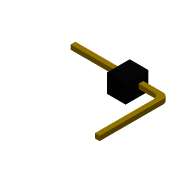
# Autodesk Inventor part: HeaderRight1
Saved by Autodesk Inventor 2015 (Build 190159000, 159)
## iProperties
Created: 2014-08-02
Part Number: HeaderRight1
Material: Generic
Document SubType Name: Modeling
Designer: david
Density: 1 g/cm^3
Appearance: Black
Author: david
Autodesk Inventor part; units mm, degrees
ref_plane "YZ Plane" through (0, 0, 0) normal (1, 0, 0) x (0, 1, 0)
ref_plane "XZ Plane" through (0, 0, 0) normal (0, 1, 0) x (-1, 0, 0)
sketch "Sketch1" plane through (0, 0, 0) normal (0, 1, 0) x (-1, 0, 0)
  line L0 (2.5467, 7.6401) -> (1.9117, 7.6401)
  line L1 (1.9117, 7.6401) -> (1.9117, -1.0276)
  line L2 (2.7055, -1.8214) -> (14.6752, -1.8214)
  line L3 (14.6752, -1.8214) -> (14.6752, -1.1864)
  line L4 (14.6752, -1.1864) -> (3.3405, -1.1864)
  line L5 (2.5467, 7.6401) -> (2.5467, -0.3926)
  line L6 (14.6752, -1.5039) -> (20.4389, -1.5039) construction
  line L7 (2.2292, 7.6401) -> (2.2292, 18.3973) construction
  line L8 (8.8332, 0.2741) -> (6.2932, 0.2741) construction
  line L9 (6.2932, 0.2741) -> (6.2932, -2.8247) construction
  line L10 (8.8332, -2.8247) -> (8.8332, 0.2741) construction
  arc A0 (2.5467, -0.3926) -> (3.3405, -1.1864) centre (3.3405, -0.3926) ccw
  arc A1 (1.9117, -1.0276) -> (2.7055, -1.8214) centre (2.7055, -1.0276) ccw
  line L11 (8.8332, -2.8247) -> (6.2932, -2.8247) construction
  dimension "d2" = 0.635
  dimension "d7" = 3.0988
  dimension "d9" = 1.778
  dimension "d10" = 7.366
  dimension "d11" = 4.064
  dimension "d12" = 5.842
  dimension "d13" = 0.7937
  constraints: 24 end point, 6 perpendicular, 4 horizontal, 4 point on circle, 4 tangent, 2 centre point, 2 midpoint, 2 vertical, 1 equal radius, 1 parallel
  measures "d2" distance of L0.start L0.end
  measures "d7" distance of L10.start L8.start
  measures "d9" distance between parallel lines of L8 L6
  measures "d10" distance between parallel lines of L8 L0
  measures "d11" distance between parallel lines of L9 L7
  measures "d12" distance between parallel lines of L10 L3
  measures "d13" radius of A0
extrude "Extrusion1" add sketch "Sketch1" along normal mid plane 0.635
ref_plane "Work Plane1" through (-5.4042, -0.3175, 7.6401) normal (-1, 0, 0) x (0, 0, 1)
sketch "Sketch2" plane through (-5.4042, -0.3175, 7.6401) normal (-1, 0, 0) x (0, 0, 1)
  line L0 (-8.8265, 0) -> (-8.8265, 0.635) projected
  line L1 (-9.4615, 0.635) -> (-8.8265, 0.635) projected
  line L2 (-9.4615, 0) -> (-9.4615, 0.635) projected
  line L3 (-8.8265, 0) -> (-9.4615, 0) projected
  line L4 (-7.0485, -0.9525) -> (-10.1473, -0.9525)
  line L5 (-10.1473, -0.9525) -> (-10.1473, 1.5875)
  line L6 (-10.1473, 1.5875) -> (-7.0485, 1.5875)
  line L7 (-7.0485, 1.5875) -> (-7.0485, -0.9525)
  line L8 (-9.144, 0) -> (-9.144, -1.4837) construction
  line L9 (-11.684, 0) -> (-11.684, -1.596) construction
  line L10 (-14.224, 0) -> (-14.224, -1.596) construction
  line L11 (-9.4615, 0.3175) -> (-12.8271, 0.3175) construction
  point P0 (-7.6401, 0.3175)
  point P1 (-10.1473, 0.3175)
  dimension "d17" = 3.0988
  dimension "d18" = 1.778
  dimension "d19" = 2.54
  constraints: 16 end point, 3 midpoint, 3 vertical, 2 horizontal, 2 parallel, 1 perpendicular, 1 point on line
  measures "d17" distance between parallel lines of L5 L7
  measures "d18" distance between parallel lines of L7 L0
  measures "d19" distance of L4.end L5.end
extrude "Extrusion2" add sketch "Sketch2" along normal blind 2.54
body "Solid1"
